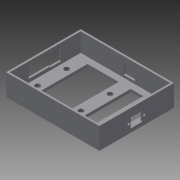
# Autodesk Inventor part: Pi Case Bottom V 01
Saved by Autodesk Inventor 2016 (Build 200138000, 138)
## iProperties
Created: 2015-03-20
Part Number: Pi Case Bottom V 01
Material: Generic
Document SubType Name: Modeling
Designer: steele
Density: 1 g/cm^3
Appearance: Default
Author: steele
Autodesk Inventor part; units mm, degrees
ref_plane "YZ Plane" through (0, 0, 0) normal (1, 0, 0) x (0, 1, 0)
ref_plane "XZ Plane" through (0, 0, 0) normal (0, 1, 0) x (-1, 0, 0)
ref_plane "XY Plane" through (0, 0, 0) normal (0, 0, 1) x (1, 0, 0)
sketch "Sketch1" plane through (0, 0, 0) normal (0, 0, 1) x (1, 0, 0)
  line L0 (-75, -60) -> (75, -60)
  line L1 (75, -60) -> (75, 60)
  line L2 (75, 60) -> (-75, 60)
  line L3 (-75, 60) -> (-75, -60)
  line L4 (-75, -60) -> (75, 60) construction
  line L5 (75, -60) -> (-75, 60) construction
  point P0 (0, 0)
  dimension "d0" = 150
  dimension "d1" = 120
  constraints: 12 end point, 2 midpoint, 2 parallel, 1 horizontal, 1 perpendicular
  measures "d0" distance of L0.start L0.end
  measures "d1" distance of L2.end L0.start
extrude "Extrusion1" add sketch "Sketch1" against normal blind 4.5
sketch "Sketch2" plane through (0, 0, 0) normal (0, 0, 1) x (1, 0, 0)
  line L0 (-75, 60) -> (75, 60)
  line L1 (75, 60) -> (75, -60)
  line L2 (75, -60) -> (-75, -60)
  line L3 (-75, -60) -> (-75, 60)
  line L4 (-72, 57) -> (72, 57)
  line L5 (72, 57) -> (72, -57)
  line L6 (72, -57) -> (-72, -57)
  line L7 (-72, -57) -> (-72, 57)
  point P0 (0, 0)
  dimension "d4" = 3
  dimension "d5" = 3
  dimension "d6" = 3
  dimension "d7" = 3
  constraints: 16 end point, 4 parallel, 2 horizontal, 2 perpendicular
  measures "d4" distance between parallel lines of L3 L7
  measures "d5" distance between parallel lines of L0 L4
  measures "d6" distance between parallel lines of L1 L5
  measures "d7" distance between parallel lines of L2 L6
extrude "Extrusion2" add sketch "Sketch2" along normal blind 30
sketch "Sketch3" plane through (75, -60, -4.5) normal (1, 0, 0) x (0, 0, -1)
  line L0 (-34.5, 0) -> (-34.5, 120) construction
  line L1 (-34.5, 60) -> (0.0994, 60) construction
  line L2 (-34.5, 0) -> (0, 0) construction
  line L3 (-17.25, 0) -> (-17.25, 120) construction
  line L4 (0, 120) -> (-34.5, 120) construction
  line L5 (-14, 0) -> (-14, 120) construction
  line L6 (-34.5, 47.5) -> (0, 47.5) construction
  line L7 (0, 0) -> (0, 120) construction
  line L8 (-34.5, 3) -> (-34.5, 117) construction
  line L9 (-34.5, 72.5) -> (0, 72.5) construction
  circle A0 centre (-14, 47.5) radius 2
  circle A1 centre (-14, 72.5) radius 2
  line L10 (-6, 50.5) -> (-6, 69.5)
  line L11 (-6, 69.5) -> (-22, 69.5)
  line L12 (-22, 69.5) -> (-22, 50.5)
  line L13 (-22, 50.5) -> (-6, 50.5)
  line L14 (-6, 50.5) -> (-22, 69.5) construction
  line L15 (-6, 69.5) -> (-22, 50.5) construction
  point P0 (-14, 60)
  dimension "d14" = 12.5
  dimension "d15" = 12.5
  dimension "d16" = 4
  dimension "d66" = 19
  dimension "d67" = 16
  constraints: 22 end point, 10 point on line, 6 midpoint, 4 parallel, 2 centre point, 2 horizontal, 2 perpendicular, 1 equal radius
  measures "d14" distance between parallel lines of L9 L1
  measures "d15" distance between parallel lines of L6 L1
  measures "d16" diameter of A0
  measures "d66" distance of L10.start L10.end
  measures "d67" distance of L11.end L10.end
sketch "Sketch5" plane through (0, 0, -4.5) normal (0, 0, -1) x (-1, 0, 0)
  line L0 (-75, -9.5) -> (-75, 9.5) construction
  line L1 (-75, 0) -> (75, 0) construction
  line L2 (75, -60) -> (75, 60) construction
  line L3 (-75, -60) -> (75, -60) construction
  line L4 (60.95, -60) -> (60.95, 60) construction
  line L5 (-75, 60) -> (75, 60) construction
  line L6 (-8.95, -60) -> (-8.95, 60) construction
  line L7 (72, 57) -> (72, -57) projected
  line L8 (72, -23.375) -> (-72, -23.375) construction
  line L9 (-72, -57) -> (-72, 57) construction
  line L10 (72, 23.375) -> (-72, 23.375) construction
  circle A0 centre (60.95, -23.375) radius 4
  circle A1 centre (-8.95, -23.375) radius 4
  circle A2 centre (-8.95, 23.375) radius 4
  circle A3 centre (60.95, 23.375) radius 4
  point P0 (0, 0)
  dimension "d20" = 11.05
  dimension "d21" = 69.9
  dimension "d22" = 23.375
  dimension "d23" = 23.375
  dimension "d24" = 8
  constraints: 16 point on line, 10 end point, 4 centre point, 3 equal radius, 2 midpoint, 2 parallel, 1 horizontal, 1 perpendicular
  measures "d20" distance between parallel lines of L4 L7
  measures "d21" distance between parallel lines of L6 L4
  measures "d22" distance between parallel lines of L8 L1
  measures "d23" distance between parallel lines of L10 L1
  measures "d24" diameter of A0
extrude "Extrusion4" cut sketch "Sketch5" against normal up to next
sketch "Sketch6" plane through (-75, -60, -4.5) normal (-1, 0, 0) x (0, 0, 1)
  line L0 (27.65, 120.0448) -> (27.65, 0.3191) construction
  line L1 (8.65, 120.0448) -> (8.65, 0.3191) construction
  line L2 (34.5, 0) -> (34.5, 120) construction
  line L3 (34.5, 85.5) -> (0, 85.5) construction
  line L4 (0, 0) -> (0, 120) construction
  line L5 (34.5, 68) -> (0, 68) construction
  line L6 (0, 120) -> (34.5, 120) projected
  line L7 (34.5, 0) -> (0, 0) projected
  line L8 (27.65, 85.5) -> (8.65, 85.5)
  line L9 (8.65, 85.5) -> (8.65, 68)
  line L10 (8.65, 68) -> (27.65, 68)
  line L11 (27.65, 68) -> (27.65, 85.5)
  point P0 (4.5, 60)
  dimension "d27" = 34.5
  dimension "d28" = 68
  dimension "d29" = 6.85
  dimension "d30" = 8.65
  constraints: 16 end point, 8 point on line, 3 parallel, 2 horizontal, 2 vertical, 1 perpendicular
  measures "d27" distance between parallel lines of L3 L6
  measures "d28" distance between parallel lines of L5 L7
  measures "d29" distance between parallel lines of L2 L0
  measures "d30" distance between parallel lines of L1 L4
extrude "Extrusion5" cut sketch "Sketch6" against normal up to next
sketch "Sketch7" plane through (-75, -60, -4.5) normal (-1, 0, 0) x (0, 0, 1)
  line L0 (0, 120) -> (34.5, 120) construction
  line L1 (31, 120) -> (31, 0.0117) construction
  line L2 (10, 120) -> (10, 0) construction
  line L3 (0, 0) -> (34.5, 0) construction
  line L4 (0, 0) -> (0, 120) construction
  line L5 (34.5, 120) -> (34.5, 0) construction
  line L6 (31, 33.25) -> (10, 33.25) construction
  line L7 (31, 69.25) -> (10, 69.25) construction
  line L8 (31, 69.25) -> (10, 69.25)
  line L9 (10, 69.25) -> (10, 33.25)
  line L10 (10, 33.25) -> (31, 33.25)
  line L11 (31, 33.25) -> (31, 69.25)
  point P0 (4.5, 60)
  dimension "d33" = 10
  dimension "d34" = 3.5
  dimension "d35" = 33.25
  dimension "d36" = 69.25
  constraints: 16 end point, 7 point on line, 3 perpendicular, 2 parallel, 2 vertical, 1 horizontal
  measures "d33" distance between parallel lines of L4 L2
  measures "d34" distance between parallel lines of L5 L1
  measures "d35" distance between parallel lines of L3 L6
  measures "d36" distance between parallel lines of L7 L3
extrude "Extrusion6" cut sketch "Sketch7" against normal blind 5
sketch "Sketch8" plane through (-75, 60, -4.5) normal (0, 1, 0) x (1, 0, 0)
  line L0 (150, 0) -> (150, -34.5) construction
  line L1 (150, -22) -> (0.3989, -22) construction
  line L2 (150, -8.5) -> (0.3989, -8.5) construction
  line L3 (90, -31) -> (90, 0) construction
  line L4 (72, -31) -> (72, 0) construction
  line L5 (150, 0) -> (0, 0) construction
  line L6 (150, -34.5) -> (0, -34.5) construction
  line L7 (0, 0) -> (0, -34.5) construction
  line L8 (90, -22) -> (72, -22)
  line L9 (72, -22) -> (72, -8.5)
  line L10 (72, -8.5) -> (90, -8.5)
  line L11 (90, -8.5) -> (90, -22)
  point P0 (75, -4.5)
  dimension "d39" = 12.5
  dimension "d40" = 8.5
  dimension "d41" = 72
  dimension "d42" = 90
  constraints: 16 end point, 7 point on line, 2 horizontal, 2 parallel, 2 perpendicular, 2 vertical
  measures "d39" distance between parallel lines of L1 L6
  measures "d40" distance between parallel lines of L2 L5
  measures "d41" distance between parallel lines of L4 L7
  measures "d42" distance between parallel lines of L3 L7
extrude "Extrusion7" cut sketch "Sketch8" against normal blind 5
sketch "Sketch10" plane through (0, 0, 0) normal (0, 0, 1) x (1, 0, 0)
  point P0 (45.375, -12.375)
hole "Hole2" at (45.375, -12.375, 0) direction (0, 0, -1) diameter 2.459 depth 8.4 tip angle 120 thread size "M3x0.5" class "6H" standard "ANSI Metric M Profile"
sketch "Sketch11" plane through (0, 0, 0) normal (0, 0, 1) x (1, 0, 0)
  point P0 (45.375, 12.375)
hole "Hole4" at (45.375, 12.375, 0) direction (0, 0, -1) diameter 2.459 depth 8.4 tip angle 120 thread size "M3x0.5" class "6H" standard "ANSI Metric M Profile"
extrude "Extrusion8" cut sketch "Sketch3" against normal up to next
sketch "Sketch12" plane through (0, 0, -4.5) normal (0, 0, -1) x (-1, 0, 0)
  line L0 (72, -57) -> (72, 57) construction
  line L1 (72, 0) -> (-72, 0) construction
  line L2 (-72, -57) -> (-72, 57) construction
  line L3 (72, -57) -> (-72, -57) construction
  line L4 (26, -57) -> (26, 57) construction
  line L5 (-28.548, -57) -> (-28.548, 57) construction
  line L6 (-72, 57) -> (72, 57) construction
  circle A0 centre (-8.95, 23.375) radius 4 construction
  line L7 (-12.95, 23.375) -> (-12.95, -23.375) construction
  circle A1 centre (-8.95, -23.375) radius 4 construction
  circle A2 centre (-45.375, -12.375) radius 1.2295 construction
  line L8 (-44.1455, -12.375) -> (-44.1455, 12.375) construction
  circle A3 centre (-45.375, 12.375) radius 1.2295 construction
  line L9 (-4.95, -23.375) -> (-4.95, 23.375) construction
  line L10 (56.95, 23.375) -> (56.95, -23.375) construction
  circle A4 centre (60.95, -23.375) radius 4 construction
  line L11 (51, 47) -> (51, -47)
  line L12 (51, -47) -> (1, -47)
  line L13 (1, -47) -> (1, 47)
  line L14 (1, 47) -> (51, 47)
  line L15 (51, 47) -> (1, -47) construction
  line L16 (51, -47) -> (1, 47) construction
  line L17 (-18.548, 47) -> (-18.548, -47)
  line L18 (-18.548, -47) -> (-38.548, -47)
  line L19 (-38.548, -47) -> (-38.548, 47)
  line L20 (-38.548, 47) -> (-18.548, 47)
  line L21 (-18.548, 47) -> (-38.548, -47) construction
  line L22 (-18.548, -47) -> (-38.548, 47) construction
  line L23 (-46.6045, -12.375) -> (-46.6045, 12.375) construction
  line L24 (-59.3025, -57) -> (-59.3025, 57) construction
  line L25 (-53.8025, 47) -> (-53.8025, -47)
  line L26 (-53.8025, -47) -> (-64.8025, -47)
  line L27 (-64.8025, -47) -> (-64.8025, 47)
  line L28 (-64.8025, 47) -> (-53.8025, 47)
  line L29 (-53.8025, 47) -> (-64.8025, -47) construction
  line L30 (-53.8025, -47) -> (-64.8025, 47) construction
  point P0 (0, 0)
  point P1 (26, 0)
  point P2 (-28.548, 0)
  point P3 (-59.3025, 0)
  dimension "d71" = 15.598
  dimension "d72" = 30.95
  dimension "d73" = 94
  dimension "d74" = 50
  dimension "d75" = 94
  dimension "d76" = 20
  dimension "d77" = 12.698
  dimension "d78" = 94
  dimension "d79" = 11
  constraints: 54 end point, 11 midpoint, 9 parallel, 8 point on circle, 5 point on line, 4 perpendicular, 4 tangent, 4 vertical, 1 horizontal alignment, 1 other
  measures "d71" distance between parallel lines of L5 L7
  measures "d72" distance between parallel lines of L4 L10
  measures "d73" distance of L11.start L11.end
  measures "d74" distance of L13.end L11.start
  measures "d75" distance of L17.start L17.end
  measures "d76" distance of L19.end L17.start
  measures "d77" distance between parallel lines of L24 L23
  measures "d78" distance of L25.start L25.end
  measures "d79" distance of L27.end L25.start
extrude "Extrusion9" cut sketch "Sketch12" against normal up to next
body "Solid1"
